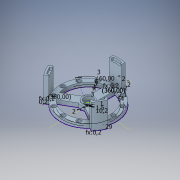
# Autodesk Inventor part: ShaftHolder
Saved by Autodesk Inventor 2018.3 (Build 223284000, 284)
## iProperties
Created: 2018-07-23
Part Number: ShaftHolder
Material: Generisch
Document SubType Name: Modeling
Designer: JochenAlt
Density: 1 g/cm^3
Appearance: Vorgabe
Author: JochenAlt
Autodesk Inventor part; units mm, degrees
ref_plane "YZ Plane" through (0, 0, 0) normal (1, 0, 0) x (0, 1, 0)
ref_plane "XZ Plane" through (0, 0, 0) normal (0, 1, 0) x (-1, 0, 0)
ref_plane "XY Plane" through (0, 0, 0) normal (0, 0, 1) x (1, 0, 0)
sketch "Skizze1" plane through (0, 0, 0) normal (0, 0, 1) x (1, 0, 0)
  circle A0 centre (0, 0) radius 29 construction
  circle A1 centre (0, 0) radius 5.1
  circle A2 centre (0, 0) radius 6.6
  circle A3 centre (0, 0) radius 4.1
  line L0 (0, 49.6) -> (0, -45.6) construction
  line L1 (-48.5477, 0) -> (48.5477, 0) construction
  line L2 (-5, 25.5147) -> (-5, 6.9971)
  line L3 (0, 0) -> (-28.9685, 16.725) construction
  line L4 (-24.5964, -8.4272) -> (-8.5597, 0.8316)
  arc A4 (-5, 6.9971) -> (-8.5597, 0.8316) centre (0, 0) ccw
  arc A5 (-5, 25.5147) -> (-24.5964, -8.4272) centre (0, 0) ccw
  line L5 (19.5964, -17.0875) -> (3.5597, -7.8287)
  arc A6 (-19.5964, -17.0875) -> (19.5964, -17.0875) centre (0, 0) ccw
  line L6 (-19.5964, -17.0875) -> (-3.5597, -7.8287)
  arc A7 (-3.5597, -7.8287) -> (3.5597, -7.8287) centre (0, 0) ccw
  line L7 (5, 25.5147) -> (5, 6.9971)
  arc A8 (24.5964, -8.4272) -> (5, 25.5147) centre (0, 0) ccw
  line L8 (24.5964, -8.4272) -> (8.5597, 0.8316)
  arc A9 (8.5597, 0.8316) -> (5, 6.9971) centre (0, 0) ccw
  circle A10 centre (0, 29) radius 2.1
  circle A11 centre (-14.5, 25.1147) radius 2.1
  circle A12 centre (-25.1147, 14.5) radius 2.1
  circle A13 centre (-29, 0) radius 2.1
  circle A14 centre (-25.1147, -14.5) radius 2.1
  circle A15 centre (-14.5, -25.1147) radius 2.1
  circle A16 centre (0, -29) radius 2.1
  circle A17 centre (14.5, -25.1147) radius 2.1
  circle A18 centre (25.1147, -14.5) radius 2.1
  circle A19 centre (29, 0) radius 2.1
  circle A20 centre (25.1147, 14.5) radius 2.1
  circle A21 centre (0, 0) radius 32
  circle A22 centre (14.5, 25.1147) radius 2.1
  line L9 (-5, 31.607) -> (-5, 35.6511)
  line L10 (5, 31.607) -> (5, 35.6511)
  line L11 (-29.8724, -11.4734) -> (-33.3747, -13.4954)
  line L12 (24.8724, -20.1336) -> (28.3747, -22.1557)
  line L13 (29.8724, -11.4734) -> (33.3747, -13.4954)
  line L14 (-24.8724, -20.1336) -> (-28.3747, -22.1557)
  arc A23 (5, 33.6303) -> (-5, 33.6303) centre (0, 0) ccw
  arc A24 (-31.6247, -12.485) -> (-26.6247, -21.1453) centre (0, 0) ccw
  arc A25 (26.6247, -21.1453) -> (31.6247, -12.485) centre (0, 0) ccw
  line L15 (-30.5416, -9.5503) -> (-34.0819, -11.5943)
  line L16 (-23.5416, -21.6747) -> (-27.0819, -23.7186)
  line L17 (-7, 31.225) -> (-7, 35.3129)
  line L18 (7, 31.225) -> (7, 35.3129)
  line L19 (23.5416, -21.6747) -> (27.0819, -23.7186)
  line L20 (30.5416, -9.5503) -> (34.0819, -11.5943)
  arc A26 (7, 35.3129) -> (-7, 35.3129) centre (0, 0) ccw
  arc A27 (-34.0819, -11.5943) -> (-27.0819, -23.7186) centre (0, 0) ccw
  arc A28 (27.0819, -23.7186) -> (34.0819, -11.5943) centre (0, 0) ccw
  line L21 (-25.1147, -14.5) -> (0, 0) construction
  circle A29 centre (0, 29) radius 2
  circle A30 centre (14.5, 25.1147) radius 2
  circle A31 centre (25.1147, 14.5) radius 2
  circle A32 centre (29, 0) radius 2
  circle A33 centre (25.1147, -14.5) radius 2
  circle A34 centre (14.5, -25.1147) radius 2
  circle A35 centre (0, -29) radius 2
  circle A36 centre (-14.5, -25.1147) radius 2
  circle A37 centre (-25.1147, -14.5) radius 2
  circle A38 centre (-29, 0) radius 2
  circle A39 centre (-25.1147, 14.5) radius 2
  circle A40 centre (-14.5, 25.1147) radius 2
  line L22 (-31.375, -12.5718) -> (-29.7993, -11.6621)
  line L23 (-26.575, -20.8856) -> (-24.9993, -19.9759)
  arc A41 (-31.375, -12.5718) -> (-26.575, -20.8856) centre (0, 0) ccw
  arc A42 (26.575, -20.8856) -> (31.375, -12.5718) centre (0, 0) ccw
  line L24 (31.375, -12.5718) -> (29.7993, -11.6621)
  line L25 (26.575, -20.8856) -> (24.9993, -19.9759)
  arc A43 (4.8, 33.4536) -> (-4.8, 33.4613) centre (-0.027, 0) ccw
  line L26 (-4.8, 33.4613) -> (-4.8, 31.638)
  line L27 (4.8, 33.4536) -> (4.8, 31.638)
  point P0 (0, -8.6)
  dimension "d1" = 29
  dimension "d2" = 10.2
  dimension "d12" = 1
  dimension "d17" = 60
  dimension "d20" = 5
  dimension "d23" = 360
  dimension "d32" = 360
  dimension "d35" = 3
  dimension "d36" = 3
  dimension "d41" = 2
  dimension "d43" = 2
  dimension "d44" = 2
  dimension "d63" = 1.5
  dimension "d66" = 2
  dimension "d67" = 2.1
  dimension "d68" = 4
  dimension "d71" = 360
  dimension "d75" = 0.2
  dimension "d76" = 0.2
  dimension "d79" = 0.2
  dimension "d80" = 0.2
  constraints: 52 end point, 43 centre point, 39 point on circle, 12 coincident, 10 point on line, 6 collinear, 6 equal radius, 5 parallel, 3 vertical, 1 midpoint, 119 other
  measures "d1" radius of A0
  measures "d2" diameter of A1
  measures "d12" radial gap between concentric circles of A1 A3
  measures "d17" angle of L0 L3
  measures "d20" distance between parallel lines of L0 L2
  measures "d35" radial gap between concentric circles of A5 A0
  measures "d43" radial gap between concentric circles of A26 A23
  measures "d44" distance between parallel lines of L17 L9
  measures "d63" radial gap between concentric circles of A2 A1
  measures "d66" radial gap between concentric circles of A7 A2
  measures "d67" radius of A10
  measures "d68" diameter of A29
  measures "d75" distance between parallel lines of L14 L23
  measures "d76" radial gap between concentric circles of A24 A41
  measures "d79" distance between parallel lines of L9 L26
  measures "d80" distance between parallel lines of L12 L25
extrude "Extrusion1" add sketch "Skizze1" along normal blind 1.5 contours A1 | A2 | A10 | A11 | A12 | A13 | A14 | A15 | A16 | A17 | A18 | A19 | A20 | A21 | A21 L10 A26 L18 | L20 A28 L13 A21 | A21 L27 A43 L26 L9 A23 L10 | L13 A25 L12 A21 L25 A42 L24 | A21 L26 A43 L27 | A23 L9 A26 L10 | L24 A42 L25 A21 | L13 A28 L12 A25 | L9 A21 L17 A26 | L12 A28 L19 A21 | A21 L11 A27 L15 | L16 A27 L14 A21 | A21 L22 A41 L23 L14 A24 L11 | A21 L23 A41 L22 | A24 L14 A27 L11 | A22 | A29 | A30 | A31 | A32 | A33 | A34 | A35 | A36 | A37 | A38 | A39 | A40
extrude "Extrusion2" add sketch "Skizze1" along normal blind 3 from surface at 1.5 contours A2 | A21 | A21 L10 A26 L18 | L20 A28 L13 A21 | A21 L27 A43 L26 L9 A23 L10 | L13 A25 L12 A21 L25 A42 L24 | A21 L26 A43 L27 | A23 L9 A26 L10 | L24 A42 L25 A21 | L13 A28 L12 A25 | L9 A21 L17 A26 | L12 A28 L19 A21 | A21 L11 A27 L15 | L16 A27 L14 A21 | A21 L22 A41 L23 L14 A24 L11 | A21 L23 A41 L22 | A24 L14 A27 L11
extrude "Extrusion12" add sketch "Skizze1" along normal blind 1 from surface at 4.5 contours A2
extrude "Extrusion6" add sketch "Skizze1" along normal blind 21 from surface at 4.5 contours A21 L10 A26 L18 | L20 A28 L13 A21 | A21 L27 A43 L26 L9 A23 L10 | L13 A25 L12 A21 L25 A42 L24 | A21 L26 A43 L27 | A23 L9 A26 L10 | L24 A42 L25 A21 | L13 A28 L12 A25 | L9 A21 L17 A26 | L12 A28 L19 A21 | A21 L11 A27 L15 | L16 A27 L14 A21 | A21 L22 A41 L23 L14 A24 L11 | A21 L23 A41 L22 | A24 L14 A27 L11
chamfer "Fase1" distance 0.5 angle 45 12 edges at (-27.2147, -14.5, 4.5) (-31.1, 0, 4.5) (-27.2147, 14.5, 4.5) (-16.6, 25.1147, 4.5) (-2.1, 29, 4.5) (12.4, 25.1147, 4.5) (23.0147, 14.5, 4.5) (26.9, 0, 4.5) (-16.6, -25.1147, 4.5) (-2.1, -29, 4.5) (12.4, -25.1147, 4.5) (23.0147, -14.5, 4.5)
extrude "Extrusion7" add sketch "Skizze1" along normal blind 3 from surface at 25.5 contours A21 L10 A26 L18 | L20 A28 L13 A21 | A23 L9 A26 L10 | L13 A28 L12 A25 | L9 A21 L17 A26 | L12 A28 L19 A21 | A21 L11 A27 L15 | L16 A27 L14 A21 | A24 L14 A27 L11
extrude "Extrusion8" add sketch "Skizze1" along normal blind 3 from surface at 25.5 separate body contours A2 | A21 | A21 L26 A43 L27 | L24 A42 L25 A21 | A21 L23 A41 L22
extrude "Extrusion9" add sketch "Skizze1" along normal blind 1.5 from surface at 28.5 contours A1 | A2 | A10 | A11 | A12 | A13 | A14 | A15 | A16 | A17 | A18 | A19 | A20 | A21 | A21 L10 A26 L18 | L20 A28 L13 A21 | A21 L27 A43 L26 L9 A23 L10 | L13 A25 L12 A21 L25 A42 L24 | A21 L26 A43 L27 | A23 L9 A26 L10 | L24 A42 L25 A21 | L13 A28 L12 A25 | L9 A21 L17 A26 | L12 A28 L19 A21 | A21 L11 A27 L15 | L16 A27 L14 A21 | A21 L22 A41 L23 L14 A24 L11 | A21 L23 A41 L22 | A24 L14 A27 L11 | A22 | A29 | A30 | A31 | A32 | A33 | A34 | A35 | A36 | A37 | A38 | A39 | A40 bodies 2
extrude "Extrusion11" add sketch "Skizze1" against normal blind 1 from surface at 25.5 contours A2 bodies 2
chamfer "Fase2" distance 0.5 angle 45 13 edges at (23.0147, 14.5, 25.5) (12.4, 25.1147, 25.5) (26.9, 0, 25.5) (23.0147, -14.5, 25.5) (12.4, -25.1147, 25.5) (-2.1, -29, 25.5) (-16.6, 25.1147, 25.5) (-27.2147, 14.5, 25.5) (-31.1, 0, 25.5) (-16.6, -25.1147, 25.5) (-27.2147, -14.5, 25.5) (-2.1, 29, 25.5) (-5.1, 0, 25.5)
extrude "Extrusion13" [suppressed]
